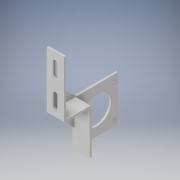
# Autodesk Inventor part: Motorhalterung_Links
Saved by Autodesk Inventor 2017 (Build 210142000, 142)
## iProperties
Part Number: Motorhalterung_Links
Material: Generisch
Document SubType Name: Modeling
Designer: Dima
Density: 1 g/cm^3
Appearance: Vorgabe
Author: Dima
Autodesk Inventor part; units mm, degrees
ref_plane "YZ Plane" through (0, 0, 0) normal (1, 0, 0) x (0, 1, 0)
ref_plane "XZ Plane" through (0, 0, 0) normal (0, 1, 0) x (-1, 0, 0)
ref_plane "XY Plane" through (0, 0, 0) normal (0, 0, 1) x (1, 0, 0)
sketch "Skizze1" plane through (0, 0, 0) normal (0, 1, 0) x (-1, 0, 0)
  line L0 (12.5, 72.5) -> (-12.5, 72.5)
  line L1 (-12.5, 72.5) -> (-12.5, -72.5)
  line L2 (-12.5, -72.5) -> (12.5, -72.5)
  line L3 (12.5, -72.5) -> (12.5, 72.5)
  point P0 (0, 0)
  point P1 (0, 72.5)
  point P2 (-12.5, 0)
  dimension "d0" = 25
  dimension "d1" = 145
  constraints: 8 end point, 2 midpoint, 2 parallel, 1 horizontal, 1 horizontal alignment, 1 perpendicular, 1 vertical alignment
  measures "d0" distance between parallel lines of L3 L1
  measures "d1" distance between parallel lines of L2 L0
extrude "Extrusion1" add sketch "Skizze1" along normal blind 100
sketch "Skizze2" plane through (12.5, 0, 72.5) normal (1, 0, 0) x (0, 0, -1)
  line L0 (0, 0) -> (145, 0) construction
  line L1 (145, 0) -> (145, 100) construction
  line L2 (0, 100) -> (145, 100) construction
  line L3 (0, 0) -> (0, 100) construction
  line L4 (0, 100) -> (80, 100)
  line L5 (80, 100) -> (80, 40)
  line L6 (80, 40) -> (0, 40)
  line L7 (0, 40) -> (0, 100)
  point P0 (72.5, 0)
  dimension "d4" = 80
  dimension "d5" = 60
  constraints: 8 end point, 2 parallel, 1 horizontal, 1 perpendicular
  measures "d4" distance of L5.end L6.end
  measures "d5" distance of L4.end L5.end
extrude "Extrusion2" cut sketch "Skizze2" against normal through all
sketch "Skizze3" plane through (12.5, 0, 72.5) normal (1, 0, 0) x (0, 0, -1)
  line L0 (80, 100) -> (80, 40) construction
  line L1 (80, 40) -> (0, 40) construction
  line L2 (0, 0) -> (0, 40) construction
  line L3 (0, 0) -> (145, 0) construction
  line L4 (145, 0) -> (145, 100) construction
  line L5 (80, 100) -> (145, 100) construction
  line L6 (0, 40) -> (80, 40)
  line L7 (80, 40) -> (80, 3)
  line L8 (80, 3) -> (0, 3)
  line L9 (0, 3) -> (0, 40)
  line L10 (80, 100) -> (145, 100)
  line L11 (145, 100) -> (145, 40)
  line L12 (145, 40) -> (80, 40)
  line L13 (80, 40) -> (80, 100)
  line L14 (145, 0) -> (83, 0)
  line L15 (83, 0) -> (83, 37)
  line L16 (83, 37) -> (145, 37)
  line L17 (145, 37) -> (145, 0)
  point P0 (72.5, 0)
  dimension "d8" = 3
  dimension "d9" = 3
  dimension "d10" = 3
  constraints: 24 end point, 6 parallel, 3 horizontal, 3 perpendicular
  measures "d8" distance between parallel lines of L3 L8
  measures "d9" distance between parallel lines of L16 L12
  measures "d10" distance between parallel lines of L7 L15
extrude "Extrusion3" cut sketch "Skizze3" against normal blind 22
sketch "Skizze4" plane through (-9.5, 0, 72.5) normal (1, 0, 0) x (0, 0, -1)
  line L0 (0, 40) -> (80, 40) construction
  line L1 (0, 3) -> (0, 40) construction
  line L2 (80, 3) -> (0, 3) construction
  line L3 (80, 40) -> (80, 3) construction
  line L4 (80, 40) -> (80, 3)
  line L5 (80, 3) -> (45, 3)
  line L6 (45, 3) -> (80, 40)
  line L7 (80, 3) -> (0, 3) projected
  line L8 (145, 0) -> (83, 0) construction
  line L9 (145, 37) -> (145, 0) construction
  line L10 (83, 37) -> (145, 37) construction
  line L11 (83, 0) -> (83, 37) construction
  line L12 (118, 37) -> (83, 3)
  line L13 (83, 37) -> (118, 37)
  line L14 (83, 3) -> (83, 37)
  line L15 (45, 3) -> (0, 3)
  line L16 (0, 0) -> (0, 40) projected
  line L17 (0, 40) -> (0, 3)
  line L18 (0, 40) -> (80, 40)
  line L19 (83, 3) -> (83, 0)
  line L20 (145, 0) -> (0, 0) projected
  line L21 (83, 0) -> (145, 0)
  line L22 (145, 37) -> (145, 0) projected
  line L23 (145, 0) -> (145, 37)
  line L24 (145, 37) -> (118, 37)
  point P0 (72.5, 0)
  dimension "d13" = 35
  dimension "d14" = 35
  constraints: 26 end point, 5 collinear, 4 perpendicular, 3 point on line, 2 vertical, 1 horizontal alignment
  measures "d13" distance of L2.start L5.end
  measures "d14" distance of L10.start L12.start
extrude "Extrusion4" cut sketch "Skizze4" against normal through all contours L6 L7 L16 L18 | L24 L22 L20 L19 L12
sketch "Skizze5" plane through (-9.5, 0, 72.5) normal (1, 0, 0) x (0, 0, -1)
  line L0 (80, 40) -> (80, 100) construction
  line L1 (145, 40) -> (80, 40) construction
  line L2 (145, 100) -> (145, 40) construction
  line L3 (80, 100) -> (145, 100) construction
  line L4 (80, 40) -> (80, 100) construction
  line L5 (80, 70) -> (145, 70) construction
  line L6 (145, 100) -> (145, 40) construction
  line L7 (80, 100) -> (145, 100) construction
  line L8 (112.5, 100) -> (112.5, 40) construction
  line L9 (145, 40) -> (80, 40) construction
  point P0 (72.5, 0)
  point P1 (88.5, 94)
  point P2 (136.5, 94)
  point P3 (136.5, 46)
  point P4 (88.5, 46)
  dimension "d17" = 48
  dimension "d18" = 48
  constraints: 4 end point, 4 midpoint, 2 horizontal alignment, 2 symmetric about line, 2 vertical alignment
  measures "d17" distance of point (136.5, 94) point (88.5, 94)
  measures "d18" distance of point (88.5, 46) point (88.5, 94)
hole "Bohrung1" at (-9.5, 94, -16) at (-9.5, 94, -64) at (-9.5, 46, -64) at (-9.5, 46, -16) direction (-1, 0, 0) diameter 4.5 end through all
sketch "Skizze6" plane through (-9.5, 0, 72.5) normal (1, 0, 0) x (0, 0, -1)
  circle A0 centre (136.5, 46) radius 2.25 projected
  circle A1 centre (88.5, 94) radius 2.25 projected
  circle A2 centre (136.5, 94) radius 2.25 projected
  circle A3 centre (88.5, 46) radius 2.25 projected
  line L0 (80, 40) -> (80, 100) projected
  line L1 (145, 40) -> (80, 40) projected
  line L2 (145, 100) -> (145, 40) projected
  line L3 (80, 100) -> (145, 100) projected
  point P0 (72.5, 0)
  point P1 (112.5, 70)
  point P2 (80, 70)
  point P3 (112.5, 100)
  constraints: 2 midpoint, 1 horizontal alignment, 1 vertical alignment
hole "Bohrung2" at (-9.5, 70, -40) direction (-1, 0, 0) diameter 40 end through all
sketch "Skizze7" plane through (12.5, 3, 72.5) normal (0, 1, 0) x (1, 0, 0)
  line L0 (0, 80) -> (0, 0) construction
  line L1 (0, 80) -> (-22, 80) construction
  line L2 (-22, 80) -> (-22, 45) construction
  line L3 (-22, 45) -> (-25, 45) construction
  line L4 (-25, 0) -> (-25, 45) construction
  line L5 (0, 0) -> (-25, 0) construction
  line L6 (-9.5, 13) -> (-9.5, 29)
  arc A0 (-9.5, 29) -> (-15.5, 29) centre (-12.5, 29) ccw
  line L7 (-15.5, 29) -> (-15.5, 13)
  arc A1 (-15.5, 13) -> (-9.5, 13) centre (-12.5, 13) ccw
  line L8 (-9.5, 53) -> (-9.5, 69)
  arc A2 (-9.5, 69) -> (-15.5, 69) centre (-12.5, 69) ccw
  line L9 (-15.5, 69) -> (-15.5, 53)
  arc A3 (-15.5, 53) -> (-9.5, 53) centre (-12.5, 53) ccw
  line L10 (0, 10) -> (-25, 10) construction
  line L11 (0, 32) -> (-25, 32) construction
  line L12 (0, 80) -> (0, 0) construction
  line L13 (-25, 0) -> (-25, 45) construction
  line L14 (0, 50) -> (-22, 50) construction
  line L15 (0, 72) -> (-22, 72) construction
  point P0 (-12.5, 72.5)
  point P1 (-12.5, 0)
  dimension "d33" = 6
  dimension "d34" = 22
  dimension "d35" = 10
  dimension "d36" = 40
  dimension "d37" = 22
  constraints: 16 end point, 12 point on line, 12 tangent, 8 point on circle, 4 centre point, 4 horizontal, 2 vertical alignment, 1 midpoint, 1 parallel, 1 vertical
  measures "d33" distance between parallel lines of L7 L6
  measures "d34" distance between parallel lines of L11 L10
  measures "d35" distance between parallel lines of L5 L10
  measures "d36" distance between parallel lines of L14 L10
  measures "d37" distance between parallel lines of L14 L15
extrude "Extrusion5" cut sketch "Skizze7" against normal through all
fillet "Rundung1" radius 2.5 4 edges at (1.5, 40, -7.5) (1.5, 37, -10.5) (0, 0, -10.5) (1.5, 3, -7.5)
equation "\"d14\" = d13"
equation "\"d18\" = d17"
equation "\"d37\" = d34"
